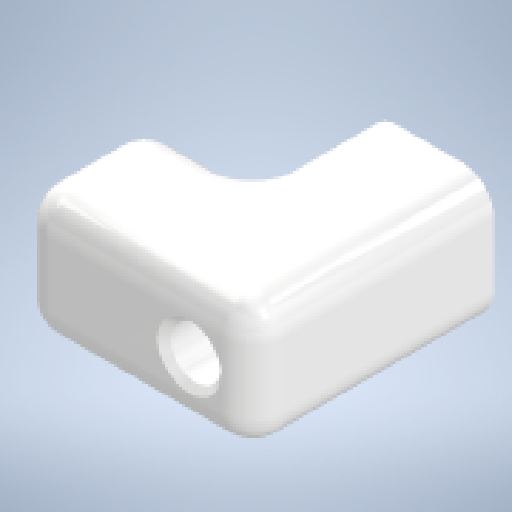
# Autodesk Inventor part: Stoper
Saved by Autodesk Inventor 2024.4 (Build 284460000, 460)
## iProperties
Created: 2026-01-11
Part Number: Stoper
Material: PVC, hart
Description: Stoper
Document SubType Name: Modeling
Designer: julia
Mass: 23.9895 g
Surface Area: 52.9425 cm^2
Volume: 18.5965 cm^3
Density: 1.29 g/cm^3
Appearance: Glatt - Weiß
DocNumber: Stoper.ipt
Folder: I60-Konstruktion\I60-Gruppe-7\Sitz\
VDS_Category: Konstruktion
Masse[kg]: 0,0008 kg
Autodesk Inventor part; units mm, degrees
ref_plane "YZ Plane" through (0, 0, 0) normal (1, 0, 0) x (0, 1, 0)
ref_plane "XZ Plane" through (0, 0, 0) normal (0, 1, 0) x (-1, 0, 0)
ref_plane "XY Plane" through (0, 0, 0) normal (0, 0, 1) x (1, 0, 0)
sketch "Skizze2" plane through (0, 0, 0) normal (0, 1, 0) x (-1, 0, 0)
  line L0 (0, 0) -> (-20, 0)
  line L1 (-20, 0) -> (-20, 20)
  line L2 (-20, 20) -> (0, 20)
  line L3 (0, 20) -> (0, 0)
  dimension "d4" = 20
  dimension "d5" = 20
  constraints: 8 end point, 2 parallel, 1 horizontal, 1 perpendicular
  measures "d4" distance of L1.end L2.end
  measures "d5" distance of L0.end L1.end
extrude "Extrusion2" add sketch "Skizze2" along normal blind 38
sketch "Skizze4" plane through (0, 0, 0) normal (-1, 0, 0) x (0, 0, 1)
  line L0 (20, 0) -> (0, 0) projected
  line L1 (0, 0) -> (20, 0)
  line L2 (20, 0) -> (20, 20)
  line L3 (20, 20) -> (0, 20)
  line L4 (0, 20) -> (0, 0)
  dimension "d8" = 20
  dimension "d9" = 20
  constraints: 8 end point, 2 parallel, 1 horizontal, 1 perpendicular
  measures "d8" distance of L3.end L2.end
  measures "d9" distance of L2.end L1.end
extrude "Extrusion3" add sketch "Skizze4" along normal blind 17
fillet "Rundung1" radius 5 14 edges at (0, 20, 10) (-17, 20, 10) (-17, 0, 10) (20, 0, 10) (1.5, 0, 20) (20, 19, 20) (20, 19, 0) (0, 29, 20) (0, 29, 0) (-8.5, 20, 20) (-8.5, 20, 0) (-17, 10, 20) (-17, 10, 0) (1.5, 0, 0)
sketch "Skizze5" plane through (0, 0, 0) normal (0, -1, 0) x (1, 0, 0)
  line L0 (0, 5) -> (0, 15) projected
  line L1 (0, 10) -> (0, 20)
  line L2 (0, 10) -> (10, 10)
  point P0 (0, 0)
  dimension "d13" = 10
  dimension "d14" = 10
  constraints: 4 end point, 1 collinear, 1 horizontal, 1 midpoint
  measures "d13" distance of L1.start L1.end
  measures "d14" distance of L1.start L2.end
hole "Bohrung1" at (10, 0, 10) direction (0, 1, 0) diameter 8 end through all countersink diameter 10 countersink angle 90
